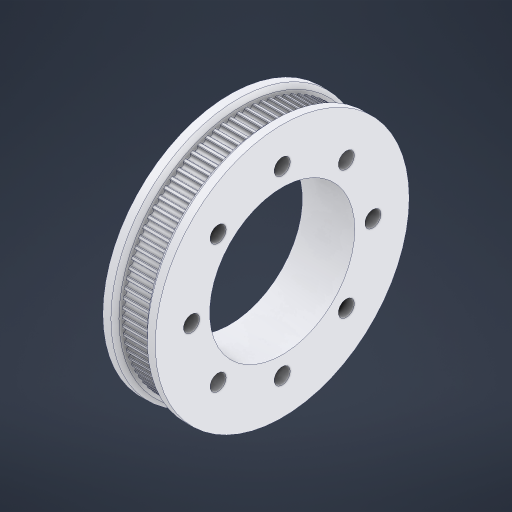
# Autodesk Inventor part: GT2 Pulley
Saved by Autodesk Inventor 2024 (Build 280153000, 153)
## iProperties
Created: 2023-10-25
Part Number: GT2 Pulley
Material: Generic
Document SubType Name: Modeling
Designer: avsar
Density: 1 g/cm^3
Appearance: PTFE
Author: avsar
Autodesk Inventor part; units mm, degrees
ref_plane "YZ Plane" through (0, 0, 0) normal (1, 0, 0) x (0, 1, 0)
ref_plane "XZ Plane" through (0, 0, 0) normal (0, 1, 0) x (-1, 0, 0)
ref_plane "XY Plane" through (0, 0, 0) normal (0, 0, 1) x (1, 0, 0)
sketch "Sketch1" plane through (0, 0, 0) normal (1, 0, 0) x (0, 1, 0)
  circle A0 centre (0, 0) radius 29.6671 construction
  circle A1 centre (0, 0) radius 28.9171 construction
  line L0 (0, 0) -> (29.6671, 0) construction
  line L1 (0, 0) -> (0, -29.6671) construction
  circle A2 centre (29.4721, 0) radius 0.555 construction
  line L2 (0, 0) -> (29.6009, -1.9815) construction
  circle A3 centre (29.4063, -1.9685) radius 0.555 construction
  circle A4 centre (29.5087, -0.704) radius 0.15 construction
  circle A5 centre (29.4899, -1.2685) radius 0.15 construction
  arc A6 (28.9171, 0) -> (29.5009, -0.5543) centre (29.4721, 0) ccw
  arc A7 (29.6587, -0.7076) -> (29.5009, -0.5543) centre (29.5087, -0.704) ccw
  arc A8 (29.6397, -1.2749) -> (29.6587, -0.7076) centre (0, 0) ccw
  arc A9 (29.4721, -1.4174) -> (29.6397, -1.2749) centre (29.4899, -1.2685) ccw
  arc A10 (29.4721, -1.4174) -> (28.8526, -1.9315) centre (29.4063, -1.9685) ccw
  arc A11 (28.8526, -1.9315) -> (28.9171, 0) centre (0, 0) ccw
  dimension "d0" = 59.3343
  dimension "d1" = -0.75
  dimension "d2" = 1.11
  dimension "d4" = 86.17
  dimension "d5" = 0.3
  constraints: 25 point on circle, 12 centre point, 8 equal radius, 8 tangent, 6 end point, 4 point on line, 1 coincident, 1 concentric, 1 horizontal, 1 perpendicular
  measures "d0" diameter of A0
  measures "d1" radial gap between concentric circles of A0 A1
  measures "d2" diameter of A2
  measures "d4" angle of L1 L2
  measures "d5" diameter of A4
extrude "Extrusion1" add sketch "Sketch1" along normal mid plane 7
pattern_circular "Circular Pattern1" count 94 over 360 about axis through (-10, 0, 0) along (1, 0, 0) of "Extrusion1"
sketch "Sketch2" plane through (0, 0, 0) normal (1, 0, 0) x (0, 1, 0)
  arc A0 (28.8526, 1.9315) -> (29.4721, 1.4174) centre (29.4063, 1.9685) ccw projected
  circle A1 centre (0, 0) radius 28.9171
  constraints: 1 coincident, 3 other
extrude "Extrusion2" add sketch "Sketch2" along normal mid plane 7
sketch "Sketch3" plane through (-3.5, 0, 0) normal (-1, 0, 0) x (0, 0, 1)
  circle A0 centre (0, 0) radius 31.5
  dimension "d13" = 63
  constraints: 1 centre point, 1 coincident
  measures "d13" diameter of A0
extrude "Extrusion3" add sketch "Sketch3" along normal blind 3
sketch "Sketch4" plane through (3.5, 0, 0) normal (1, 0, 0) x (0, 0, -1)
  circle A0 centre (0, 0) radius 31.5 projected
extrude "Extrusion4" add sketch "Sketch4" along normal blind 3
sketch "Sketch5" plane through (6.5, 0, 0) normal (1, 0, 0) x (0, 0, -1)
  circle A0 centre (0, 22.5) radius 2
  circle A1 centre (-15.9099, 15.9099) radius 2
  circle A2 centre (-22.5, 0) radius 2
  circle A3 centre (-15.9099, -15.9099) radius 2
  circle A4 centre (0, -22.5) radius 2
  circle A5 centre (15.9099, -15.9099) radius 2
  circle A6 centre (22.5, 0) radius 2
  circle A7 centre (15.9099, 15.9099) radius 2
  point P0 (0, 0)
  dimension "d18" = 4
  dimension "d19" = 22.5
  dimension "d22" = 360
  constraints: 8 centre point, 1 vertical alignment, 17 other
  measures "d18" diameter of A0
  measures "d19" distance of point (0, 0) A0.centre
extrude "Extrusion5" cut sketch "Sketch5" against normal through all
chamfer "Chamfer1" distance 1 angle 45 2 edges at (3.5, 0, 31.5) (-3.5, 0, -31.5)
sketch "Sketch6" plane through (6.5, 0, 0) normal (1, 0, 0) x (0, 0, -1)
  circle A0 centre (0, 0) radius 18
  dimension "d29" = 36
  constraints: 1 centre point, 1 coincident
  measures "d29" diameter of A0
extrude "Extrusion6" cut sketch "Sketch6" against normal through all
equation "\"d0\" = OD_"
equation "\"d1\" = H_"
equation "\"d2\" = BTD_"
equation "\"d4\" = TH_"
equation "\"d5\" = PTR_"
equation "\"d6\" = EX_"
equation "\"d11\" = EX_"
equation "\"U_\" = 0.254"
equation "\"H_\" = -0.75"
equation "\"P_\" = 2"
equation "\"BTD_\" = 1.11"
equation "\"PTR_\" = 0.3"
equation "\"EX_\" = 7"
equation "\"OD_\" = PD_ - 2 * U_"
equation "\"TH_\" = 86.170213deg"
equation "\"PD_\" = 59.842259"
body "Solid1"
